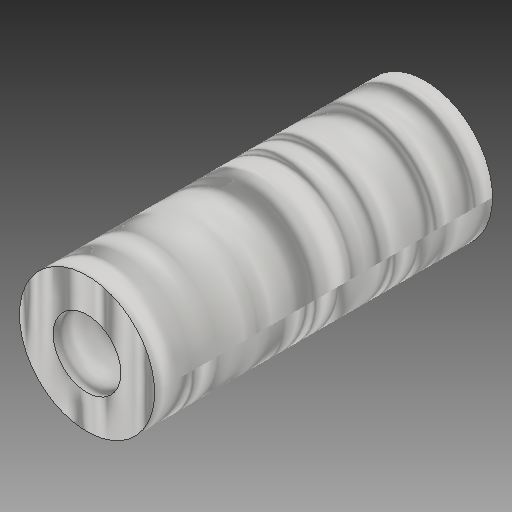
# Autodesk Inventor part: M4アルミスペーサー20
Saved by Autodesk Inventor 2017.3 (Build 213256000, 256)
## iProperties
Part Number: M4アルミスペーサー20
Material: アルミニウム 7075
Document SubType Name: Modeling
Designer: 原知也
Density: 2.81 g/cm^3
Appearance: サテン - ブラシ仕上げ 重厚
Mass: 2.25994 g
Surface Area: 8.04248 cm^2
Volume: 0.804248 cm^3
Author: 原知也
Autodesk Inventor part; units mm, degrees
ref_plane "YZ Plane" through (0, 0, 0) normal (1, 0, 0) x (0, 1, 0)
ref_plane "XZ Plane" through (0, 0, 0) normal (0, 1, 0) x (-1, 0, 0)
ref_plane "XY Plane" through (0, 0, 0) normal (0, 0, 1) x (1, 0, 0)
sketch "スケッチ1" plane through (0, 0, 0) normal (0, 0, 1) x (1, 0, 0)
  circle A0 centre (0, 0) radius 4
  dimension "d1" = 8
  constraints: 1 centre point
  measures "d1" diameter of A0
extrude "押し出し2" add sketch "スケッチ1" along normal blind 20
sketch "スケッチ2" plane through (0, 0, 0) normal (0, 0, -1) x (-1, 0, 0)
  circle A0 centre (0, 0) radius 2
  dimension "d6" = 4
  constraints: 1 centre point, 1 coincident
  measures "d6" diameter of A0
extrude "押し出し3" cut sketch "スケッチ2" against normal blind 8
sketch "スケッチ3" plane through (0, 0, 20) normal (0, 0, 1) x (1, 0, 0)
  circle A0 centre (0, 0) radius 2
  dimension "d9" = 4
  constraints: 1 centre point, 1 coincident
  measures "d9" diameter of A0
extrude "押し出し4" cut sketch "スケッチ3" against normal blind 8
